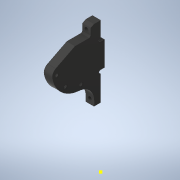
# Autodesk Inventor part: カメラ_メインフレーム
Saved by Autodesk Inventor 2020.3 (Build 243373000, 373)
## iProperties
Created: 2018-06-07
Part Number: カメラ_メインフレーム
Material: アセタール樹脂、黒
Document SubType Name: Modeling
Designer: taka
Density: 1.425 g/cm^3
Appearance: 滑らか - 黒
Mass: 5.38767 g
Surface Area: 23.5027 cm^2
Volume: 3.78082 cm^3
Category: 頭
Author: taka
Autodesk Inventor part; units mm, degrees
ref_plane "YZ Plane" through (0, 0, 0) normal (1, 0, 0) x (0, 1, 0)
ref_plane "XZ Plane" through (0, 0, 0) normal (0, 1, 0) x (-1, 0, 0)
ref_plane "XY Plane" through (0, 0, 0) normal (0, 0, 1) x (1, 0, 0)
sketch "スケッチ2" plane through (0, 0, 0) normal (0, 0, 1) x (1, 0, 0)
  line L0 (0, 0) -> (7, 0) construction
  line L1 (7, 0) -> (7, -27) construction
  line L2 (7, -27) -> (0, -27) construction
  line L3 (0, -27) -> (0, 0) construction
  circle A0 centre (2.5, -3.7) radius 1.6 construction
  circle A1 centre (2.5, -23.3) radius 1.6 construction
  line L4 (5.05, -7.5) -> (0.05, -7.5) construction
  line L5 (0.05, -7.5) -> (0.05, -19.5) construction
  line L6 (0.05, -19.5) -> (5.05, -19.5) construction
  line L7 (5.05, -19.5) -> (5.05, -7.5) construction
  line L8 (0, -7.45) -> (5.1, -7.45) construction
  line L9 (5.1, -7.45) -> (5.1, -19.55) construction
  line L10 (5.1, -19.55) -> (0, -19.55) construction
  line L11 (0, -19.55) -> (0, -7.45) construction
  line L12 (88.7886, 25.8241) -> (57.6759, -5.2886) construction
  line L13 (57.6759, -5.2886) -> (61.2114, -8.8241) construction
  line L14 (61.2114, -8.8241) -> (84.1924, 14.1569) construction
  line L15 (92.3241, 22.2886) -> (88.7886, 25.8241) construction
  line L16 (70.3953, 0.3598) -> (72.1009, 2.0653)
  circle A2 centre (100.1023, -8.117) radius 0.8
  line L17 (7, 0) -> (45.561, -10.3324) construction
  line L18 (7, -27) -> (50.4418, -38.6402) construction
  line L19 (72.4418, -38.6402) -> (106.1477, -10.3575) construction
  line L20 (106.1477, -10.3575) -> (100.2529, -4.1751) construction
  arc A3 (45.561, -10.3324) -> (81.4937, -2.447) centre (55.9138, 28.3046) ccw construction
  line L21 (72.4418, -38.6402) -> (50.4418, -38.6402) construction
  line L22 (39, -8.8) -> (34, -8.8) construction
  line L23 (34, -8.8) -> (34, -33.8) construction
  line L24 (34, -33.8) -> (39, -33.8) construction
  line L25 (39, -33.8) -> (39, -8.8) construction
  circle A4 centre (97.0056, -9.675) radius 0.8 construction
  circle A5 centre (93.6401, -10.5063) radius 0.8 construction
  circle A6 centre (90.1742, -10.5693) radius 0.8
  circle A7 centre (86.7807, -9.8609) radius 0.8 construction
  circle A8 centre (83.6295, -8.4164) radius 0.8 construction
  circle A9 centre (80.8777, -6.3081) radius 0.8
  line L26 (100.2529, -4.1751) -> (104.2516, -8.3688)
  arc A10 (81.4937, -2.447) -> (100.2529, -4.1751) centre (91.6271, 4.8718) ccw construction
  line L27 (39, -15.3) -> (34, -15.3) construction
  line L28 (34, -15.3) -> (34, -27.3) construction
  line L29 (34, -27.3) -> (39, -27.3) construction
  line L30 (39, -27.3) -> (39, -15.3) construction
  line L31 (33.95, -15.25) -> (39.05, -15.25) construction
  line L32 (39.05, -15.25) -> (39.05, -27.35) construction
  line L33 (39.05, -27.35) -> (33.95, -27.35) construction
  line L34 (33.95, -27.35) -> (33.95, -15.25) construction
  circle A11 centre (36.5, -11.5) radius 1.6 construction
  circle A12 centre (36.5, -31.1) radius 1.6 construction
  line L35 (66, -30.5) -> (71, -30.5) construction
  circle A13 centre (68.5, -34.3) radius 1.6 construction
  line L36 (66, -37) -> (71, -37) construction
  line L37 (66, -18.5) -> (66, -30.5) construction
  line L38 (65.95, -30.55) -> (65.95, -18.45) construction
  line L39 (71, -30.5) -> (71, -18.5) construction
  line L40 (66, -12) -> (66, -37) construction
  line L41 (71, -37) -> (71, -12) construction
  line L42 (71.05, -18.45) -> (71.05, -30.55) construction
  line L43 (71.05, -30.55) -> (65.95, -30.55) construction
  circle A14 centre (68.5, -14.7) radius 1.6 construction
  line L44 (71, -18.5) -> (66, -18.5) construction
  line L45 (65.95, -18.45) -> (71.05, -18.45) construction
  line L46 (71, -12) -> (66, -12) construction
  circle A15 centre (71.05, -19.5) radius 1.05 construction
  circle A16 centre (65.95, -19.5) radius 1.05 construction
  circle A17 centre (65.95, -29.5) radius 1.05 construction
  circle A18 centre (71.05, -29.5) radius 1.05 construction
  circle A19 centre (39.05, -16.3) radius 1.05 construction
  circle A20 centre (33.95, -16.3) radius 1.05 construction
  circle A21 centre (33.95, -26.3) radius 1.05 construction
  circle A22 centre (39.05, -26.3) radius 1.05 construction
  circle A23 centre (5.1, -8.5) radius 1.05 construction
  circle A24 centre (0, -8.5) radius 1.05 construction
  circle A25 centre (0, -18.5) radius 1.05 construction
  circle A26 centre (5.1, -18.5) radius 1.05 construction
  line L47 (-3, -7.45) -> (-3, -19.55) construction
  line L48 (-3, -19.55) -> (0, -27) construction
  line L49 (-3, -7.45) -> (0, 0) construction
  circle A27 centre (91.6271, 4.8718) radius 15.5 construction
  arc A28 (77.4664, -6.7113) -> (78.1043, -7.45) centre (91.6271, 4.8718) ccw construction
  line L50 (77.4664, -6.7113) -> (80.2948, -9.5397) construction
  line L51 (104.2516, -8.3688) -> (82.9591, 12.9236) construction
  line L52 (82.9591, 12.9236) -> (84.1924, 14.1569) construction
  line L53 (70.3953, 0.3598) -> (61.2114, -8.8241)
  line L54 (92.3241, 22.2886) -> (95.1525, 19.4602)
  line L55 (95.1525, 19.4602) -> (104.2516, -8.3688)
  line L56 (61.2114, -8.8241) -> (64.0398, -11.6525)
  arc A29 (90.4296, -13.3836) -> (104.2516, -8.3688) centre (91.6271, 4.8718) ccw
  line L57 (64.0398, -11.6525) -> (66.1527, -9.5397)
  arc A30 (79.9568, -9.217) -> (66.1527, -9.5397) centre (73.2238, -16.6108) ccw
  arc A31 (79.4965, -8.8227) -> (90.4296, -13.3836) centre (91.6271, 4.8718) ccw
  arc A32 (78.1501, -7.5) -> (79.4709, -8.8) centre (91.6271, 4.8718) ccw construction
  arc A33 (79.4709, -8.8) -> (79.4965, -8.8227) centre (91.6271, 4.8718) ccw
  arc A34 (78.1043, -7.45) -> (78.1501, -7.5) centre (91.6271, 4.8718) ccw construction
  line L58 (84.1924, 14.1569) -> (73.5858, 3.5503) construction
  line L59 (73.5858, 3.5503) -> (71.8887, 5.2473)
  line L60 (71.8887, 5.2473) -> (82.4953, 15.8539)
  line L61 (82.4953, 15.8539) -> (84.1924, 14.1569)
  line L62 (73.5858, 3.5503) -> (82.9591, 12.9236) construction
  line L63 (84.1924, 14.1569) -> (85.6773, 15.6418) construction
  line L64 (84.1924, 14.1569) -> (85.6773, 15.6418) construction
  arc A35 (84.1924, 14.1569) -> (85.6773, 15.6418) centre (84.9349, 14.8993) ccw
  arc A36 (72.1009, 2.0653) -> (73.5858, 3.5503) centre (72.8433, 2.8078) ccw
  arc A37 (85.6773, 15.6418) -> (84.1924, 14.1569) centre (84.9349, 14.8993) ccw construction
  line L65 (85.6773, 15.6418) -> (92.3241, 22.2886) construction
  line L66 (72.1009, 2.0653) -> (73.5858, 3.5503) construction
  arc A38 (73.5858, 3.5503) -> (72.1009, 2.0653) centre (72.8433, 2.8078) ccw construction
  line L67 (85.6773, 15.6418) -> (92.3241, 22.2886)
  point P0 (75, 8.5)
  point P1 (91.5446, -20.9171)
  point P2 (82.042, -3.1517)
  point P3 (81.2596, -2.6403)
  point P4 (55.561, -0.3324)
  point P5 (39, -14.2)
  point P6 (34, -14.2)
  point P7 (39, -28.4)
  point P8 (34, -28.4)
  dimension "d74" = 7
  dimension "d75" = 27
  dimension "d76" = 3.2
  dimension "d77" = 3.2
  dimension "d78" = 5
  dimension "d79" = 12
  dimension "d80" = 2.5
  dimension "d81" = 2.5
  dimension "d82" = 19.6
  dimension "d83" = 3.7
  dimension "d84" = 7.5
  dimension "d85" = 0.05
  dimension "d86" = 44
  dimension "d87" = 5
  dimension "d88" = 45
  dimension "d89" = 2.5
  dimension "d90" = 22
  dimension "d91" = 75
  dimension "d92" = 8.5
  dimension "d93" = 30
  dimension "d94" = 27
  dimension "d95" = 1.6
  dimension "d96" = 75
  dimension "d97" = 75
  dimension "d98" = 40
  dimension "d99" = 30
  dimension "d100" = 39
  dimension "d101" = 5
  dimension "d102" = 25
  dimension "d103" = 32
  dimension "d104" = 8.8
  dimension "d105" = 77
  dimension "d106" = 22
  dimension "d107" = 12.5
  dimension "d108" = 50
  dimension "d109" = 21
  dimension "d110" = 44
  dimension "d111" = 12
  dimension "d112" = 6.5
  dimension "d113" = 0.05
  dimension "d114" = 3.2
  dimension "d115" = 2.5
  dimension "d116" = 2.7
  dimension "d117" = 3.2
  dimension "d118" = 19.6
  dimension "d119" = 2.5
  dimension "d120" = 5
  dimension "d121" = 25
  dimension "d122" = 12
  dimension "d123" = 6.5
  dimension "d124" = 0.05
  dimension "d125" = 3.2
  dimension "d126" = 2.5
  dimension "d127" = 2.7
  dimension "d128" = 3.2
  dimension "d129" = 19.6
  dimension "d130" = 2.5
  dimension "d131" = 12
  dimension "d132" = 64
  dimension "d133" = 2.1
  dimension "d134" = 2.1
  dimension "d135" = 2.1
  dimension "d136" = 2.1
  dimension "d137" = 2.1
  constraints: 136 end point, 39 centre point, 30 point on circle, 27 point on line, 25 parallel, 24 perpendicular, 17 tangent, 15 collinear, 7 horizontal, 4 coincident, 2 midpoint, 1 vertical, 22 other
  measures "d74" distance of L18.start L2.end
  measures "d75" distance of L0.end L18.start
  measures "d76" diameter of A0
  measures "d77" diameter of A1
  measures "d78" distance of L6.end L6.start
  measures "d79" distance of L6.start L4.end
  measures "d80" distance from line of L3 A0.centre
  measures "d81" distance from line of L3 A1.centre
  measures "d82" distance of A1.centre A0.centre
  measures "d83" vertical distance of L49.end A0.centre
  measures "d84" distance between parallel lines of L0 L4
  measures "d85" distance between parallel lines of L4 L8
  measures "d86" distance of L15.start L13.end
  measures "d87" distance of L13.end L12.end
  measures "d88" angle of L0 L14
  measures "d89" distance from line of point (75, 8.5) L14
  measures "d90" distance from line of L15 point (75, 8.5)
  measures "d91" distance from line of point (75, 8.5) L3
  measures "d92" distance from line of point (75, 8.5) L0
  measures "d93" distance of point (91.545, -20.917) L16.start
  measures "d94" distance from line of L14 point (100.102, -8.117)
  measures "d95" diameter of A2
  measures "d96" angle of L1 L17
  measures "d97" angle of L18 L1
  measures "d98" radius of A3
  measures "d99" distance from line of L16 A3.centre
  measures "d100" distance from line of L21 L16.start
  measures "d101" distance of L25.start L23.end
  measures "d102" distance of L23.end L23.start
  measures "d103" distance between parallel lines of L1 L25
  measures "d104" distance between parallel lines of L22 L0
  measures "d106" distance of L19.start L18.end
  measures "d107" radius of A10
  measures "d108" angle of L3 L19
  measures "d109" distance from line of point (91.627, 4.872) L19
  measures "d110" distance of L19.start L20.start
  measures "d111" distance of L29.start L27.end
  measures "d112" distance between parallel lines of L24 L29
  measures "d113" distance between parallel lines of L27 L31
  measures "d114" diameter of A11
  measures "d115" distance from line of L23 A11.centre
  measures "d116" distance from line of L22 A11.centre
  measures "d117" diameter of A12
  measures "d118" distance of A12.centre A11.centre
  measures "d119" distance from line of L23 A12.centre
  measures "d120" distance of L41.start L40.end
  measures "d121" distance of L40.end L46.end
  measures "d122" distance of L37.end L44.end
  measures "d123" distance between parallel lines of L36 L35
  measures "d124" distance between parallel lines of L44 L45
  measures "d125" diameter of A14
  measures "d126" distance from line of L40 A14.centre
  measures "d127" distance from line of L46 A14.centre
  measures "d128" diameter of A13
  measures "d129" distance of A13.centre A14.centre
  measures "d130" distance from line of L40 A13.centre
  measures "d131" distance between parallel lines of L0 L46
  measures "d132" distance between parallel lines of L1 L41
  measures "d133" diameter of A15
  measures "d134" diameter of A16
  measures "d135" diameter of A17
  measures "d136" diameter of A18
  measures "d137" diameter of A19
extrude "押し出し2" add sketch "スケッチ2" along normal blind 5 contours L16 A36 L59 L60 L61 A35 L67 L54 L55 A29 A31 A30 L57 L56 L53
sketch "スケッチ3" plane through (85.6773, 15.6418, 0) normal (-0.7071068, 0.7071068, 0) x (-0.7071068, -0.7071068, 0)
  circle A0 centre (-6.4, 2.5) radius 1.15
  circle A1 centre (31.6, 2.5) radius 1.15
  line L0 (-9.4, 0) -> (0, 0) projected
  line L1 (-9.4, 0) -> (-9.4, 5) projected
  line L2 (34.6, 0) -> (34.6, 5) projected
  line L3 (19.2, 0) -> (34.6, 0) projected
  point P0 (71.6434, 0)
  dimension "d165" = 2.3
  dimension "d166" = 2.3
  dimension "d167" = 2.5
  dimension "d168" = 3
  dimension "d169" = 3
  dimension "d170" = 2.5
  constraints: 2 centre point
  measures "d165" diameter of A0
  measures "d166" diameter of A1
  measures "d167" distance from line of L0 A0.centre
  measures "d168" distance from line of L1 A0.centre
  measures "d169" distance from line of L2 A1.centre
  measures "d170" distance from line of L3 A1.centre
extrude "押し出し3" cut sketch "スケッチ3" against normal through all
fillet "フィレット1" radius 4 1 edges at (104.2516, -8.3688, 2.5)
sketch "スケッチ5" plane through (0, 0, 5) normal (0, 0, 1) x (1, 0, 0)
  line L0 (89.3896, 19.3541) -> (91.016, 20.9804) construction
  line L1 (103.3964, -5.7534) -> (95.1525, 19.4602) construction
  line L2 (95.9083, 17.1488) -> (92.4788, 13.7193)
  line L3 (92.4788, 13.7193) -> (99.2403, 6.9578)
  line L4 (90.2028, 20.1673) -> (100.0709, 10.2991) construction
  line L5 (92.3241, 22.2886) -> (85.6773, 15.6418) construction
  line L6 (93.2213, 14.4618) -> (93.9637, 13.7193) construction
  line L7 (93.9637, 13.7193) -> (93.2213, 12.9769) construction
  arc A0 (93.2213, 14.4618) -> (93.2213, 12.9769) centre (93.9637, 13.7193) ccw
  line L8 (93.2213, 14.4618) -> (98.519, 9.1641) construction
  line L9 (95.9083, 17.1488) -> (101.13, 11.927) construction
  line L10 (99.2403, 6.9578) -> (95.9083, 17.1488)
  point P0 (0, 0)
  point P1 (95.9083, 17.1488)
  dimension "d179" = 1.05
  dimension "d180" = 1.9
  constraints: 16 end point, 8 point on line, 4 parallel, 4 perpendicular, 2 point on circle, 1 centre point, 1 coincident, 1 collinear, 1 midpoint, 1 other
  measures "d179" distance between parallel lines of L7 L2
  measures "d180" distance from line of L6.start L4
extrude "押し出し4" cut sketch "スケッチ5" against normal up to surface (5 mm away) contours L10 L3 A0 L2
sketch "スケッチ6" plane through (61.2114, -8.8241, 0) normal (-0.7071068, 0.7071068, 0) x (-0.7071068, -0.7071068, 0)
  point P0 (37.0434, 0)
